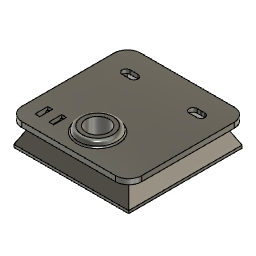
Lichtschranke Halterung (Autodesk Fusion 360 design; units mm, degrees)
Autodesk Fusion 360 part; units mm, degrees
sketch "Skizze1" plane through (0, 0, 0) normal (0, 0, 1) x (1, 0, 0)
  line L0 (0, 0) -> (43.5, 0)
  line L1 (43.5, 0) -> (43.5, 43)
  line L2 (43.5, 43) -> (0, 43)
  line L3 (0, 43) -> (0, 0)
  line L4 (-0.0245, 10) -> (43.5, 10) construction
  line L5 (21.75, 0) -> (21.75, 43) construction
  circle A0 centre (21.7377, 10) radius 4.35
  circle A1 centre (21.7377, 10) radius 7.35
  line L6 (-0.0245, 10) -> (43.5587, 10)
  line L7 (43.5587, 10) -> (43.5587, 8)
  line L8 (43.5587, 8) -> (-0.0245, 8)
  line L9 (-0.0245, 8) -> (-0.0245, 10)
  line L10 (43.5587, 12) -> (-0.0245, 12)
  line L11 (0, -23) -> (0, 20)
  line L12 (43.5, 20) -> (43.5, -23)
  line L13 (21.75, 0) -> (23.75, 0)
  line L14 (23.75, 0) -> (23.75, 43)
  line L15 (23.75, 43) -> (21.75, 43)
  line L16 (21.75, 43) -> (21.75, 0)
  line L17 (19.75, 0) -> (19.75, 43)
  line L18 (19.75, 43) -> (21.75, 43)
  line L19 (21.75, 0) -> (19.75, 0)
  dimension "d1" = 43.5
  dimension "d2" = 43
  dimension "d94" = 8.7
  dimension "d95" = 14.7
  dimension "d100" = 10
  dimension "d107" = 2
  dimension "d108" = 43.5833
  dimension "d109" = 2
  constraint horizontal L0
  constraint vertical L1
  constraint horizontal L2
  constraint vertical L3
  constraint coincident L0.start L3.end
  constraint midpoint L0 L5.start
  constraint midpoint L2 L5.end
  constraint concentric A0 A1
  constraint perpendicular L1 L4
  constraint horizontal L6
  constraint vertical L7
  constraint horizontal L8
  constraint vertical L9
  constraint symmetric L0.start L6 L11.end
  constraint symmetric L0.end L6 L12.start
  constraint symmetric L1.end L6 L12.end
  constraint symmetric L2.end L6 L11.start
  constraint symmetric L7.end L6 L10.start
  constraint symmetric L8.end L6 L10.end
  constraint horizontal L13
  constraint vertical L14
  constraint horizontal L15
  constraint vertical L16
  constraint symmetric L13.start L5 L16.end
  constraint symmetric L5 L13.end L17.start
  constraint symmetric L5 L14.end L17.end
  constraint symmetric L5 L15.end L16.start
  measures "d1" distance of L0.start L0.end
  measures "d2" distance of L0.start L2.end
  measures "d94" diameter of A0
  measures "d95" diameter of A1
  measures "d100" distance of L0.end L4.end
  measures "d107" distance of L4.start L8.end
  measures "d108" distance of L7.end L8.end
  measures "d109" distance of L5.start L13.end
extrude "Extrusion1" add sketch "Skizze1" along normal blind 1 contours L0 L3 A1 L8 L11 L17 | L0 A1 L16 L17 L19 | L3 A1 L6 L8 L11 | L0 A1 L13 L14 L16 | A0 A1 L16 L17 | A0 A1 L8 L17 | L3 A1 L6 L10 L11 | A0 A1 L6 L8 | L0 L1 A1 L8 L12 L14 | A0 A1 L14 L16 | A0 L8 L16 L17 | A0 L8 L17 | L2 L3 A1 L10 L11 L17 | A0 A1 L6 L10 | A0 L6 L8 L17 | A0 A1 L8 L14 | A0 L8 L14 L16 | L6 L8 L16 L17 | A0 A1 L10 L17 | A0 L6 L10 L17 | L1 A1 L6 L8 L12 | A0 A1 L6 L8 | A0 L8 L14 | L6 L8 L14 L16 | L6 L10 L16 L17 | L2 A1 L16 L17 L18 | A0 A1 L16 L17 | A0 L10 L17 | L1 A1 L6 L10 L12 | A0 A1 L6 L10 | A0 L6 L8 L14 | L6 L10 L14 L16 | A0 L10 L16 L17 | L2 A1 L14 L15 L16 | A0 A1 L14 L16 | L1 L2 A1 L10 L12 L14 | A0 A1 L10 L14 | A0 L6 L10 L14 | A0 L10 L14 L16 | A0 L10 L14
extrude "Extrusion2" add 1 faces at (29, 21, 1) along direction (0, 0, 1) blind 8
chamfer "Fase1" distance 4 distance2 8 4 edges at (21.75, 0, 9) (43.5, 21.5, 9) (21.75, 43, 9) (0, 21.5, 9) measured on face at (14.5, 28.6667, 9) measured on face at (14.5, 28.6667, 9) measured on face at (14.5, 28.6667, 9) measured on face at (14.5, 28.6667, 9)
sketch "Skizze2" plane through (0, 0, 9) normal (0, 0, 1) x (-1, 0, 0)
  line L0 (-39.5, -39) -> (-4, -39) construction
  line L1 (-4, -39) -> (-4, -4) construction
  line L2 (-4, -4) -> (-39.5, -4) construction
  line L3 (-39.5, -4) -> (-39.5, -39) construction
  line L4 (-39.5, -4) -> (-4, -39) construction
  line L5 (-4, -4) -> (-39.5, -39) construction
  line L6 (-44.5, -44) -> (1, -44)
  line L7 (1, -44) -> (1, 1)
  line L8 (1, 1) -> (-44.5, 1)
  line L9 (-44.5, 1) -> (-44.5, -44)
  dimension "d9" = 5
  constraint coincident L2.end L3.start
  constraint coincident L0.end L1.start
  constraint coincident L1.end L2.start
  constraint coincident L0.start L3.end
extrude "Extrusion3" add sketch "Skizze2" along normal blind 2
fillet "Abrundung1" radius 5 4 edges at (44.5, 44, 10) (-1, 44, 10) (-1, -1, 10) (44.5, -1, 10)
shell "Schale1" thickness 1.5 removed faces 1 at (29, 14.3333, 0)
sketch "Skizze7" plane through (0, 0, 11) normal (0, 0, 1) x (-1, 0, 0)
  arc A0 (-39.5, 1) -> (-44.5, -4) centre (-39.5, -4) ccw
  line L0 (-44.5, -4) -> (-44.5, -39)
  arc A1 (-44.5, -39) -> (-39.5, -44) centre (-39.5, -39) ccw
  line L1 (-39.5, -44) -> (-4, -44)
  arc A2 (-4, -44) -> (1, -39) centre (-4, -39) ccw
  line L2 (1, -39) -> (1, -4)
  arc A3 (1, -4) -> (-4, 1) centre (-4, -4) ccw
  line L3 (-4, 1) -> (-39.5, 1)
  line L4 (-6.25, -38) -> (-37.25, -38)
  line L5 (-37.25, -38) -> (-37.25, -18)
  line L6 (-37.25, -18) -> (-6.25, -18)
  line L7 (-6.25, -18) -> (-6.25, -38)
  line L8 (-21.75, -44) -> (-21.75, -32) construction
  circle A4 centre (-34.45, -35) radius 1.5
  circle A5 centre (-9.05, -35) radius 1.5
  line L9 (-4, -8.8) -> (-11.1, -8.8)
  line L10 (-11.1, -8.8) -> (-11.1, -4)
  line L11 (-11.1, -4) -> (-4, -4)
  line L12 (-4, -4) -> (-4, -8.8)
  line L13 (-5.8, -8.8) -> (-9.3, -8.8) construction
  line L14 (-9.3, -8.8) -> (-9.3, -4)
  line L15 (-9.3, -4) -> (-5.8, -4) construction
  line L16 (-5.8, -4) -> (-5.8, -8.8)
  arc A6 (-39.5, 1) -> (-44.5, -4) centre (-39.5, -4) ccw
  line L17 (-39.5, 1) -> (-4, 1)
  arc A7 (1, -4) -> (-4, 1) centre (-4, -4) ccw
  line L18 (1, -4) -> (1, -39)
  arc A8 (-4, -44) -> (1, -39) centre (-4, -39) ccw
  line L19 (-4, -44) -> (-39.5, -44)
  arc A9 (-44.5, -39) -> (-39.5, -44) centre (-39.5, -39) ccw
  line L20 (-44.5, -39) -> (-44.5, -4)
  line L21 (-39.5, -39) -> (-4, -39)
  line L22 (-4, -39) -> (-4, -4)
  line L23 (-4, -4) -> (-39.5, -4)
  line L24 (-39.5, -4) -> (-39.5, -39)
  circle A10 centre (-7.55, -35) radius 1.5
  circle A11 centre (-10.55, -35) radius 1.5
  circle A12 centre (-32.95, -35) radius 1.5
  circle A13 centre (-35.95, -35) radius 1.5
  line L25 (-32.9776, -36.4997) -> (-35.9499, -36.5)
  line L26 (-32.9776, -33.5003) -> (-35.9499, -33.5)
  line L27 (-7.5499, -36.5) -> (-10.55, -36.5)
  line L28 (-7.5501, -33.5) -> (-10.55, -33.5)
  dimension "d58" = 31
  dimension "d59" = 20
  dimension "d60" = 6
  dimension "d61" = 2.8
  dimension "d62" = 2.8
  dimension "d63" = 3
  dimension "d64" = 3
  dimension "d65" = 3
  dimension "d66" = 3
  dimension "d69" = 5
  dimension "d70" = 5
  dimension "d73" = 4.8
  dimension "d74" = 7.1
  dimension "d86" = 3.5
  dimension "d87" = 4.8
  dimension "d90" = 3
  dimension "d91" = 3
  dimension "d92" = 3
  dimension "d93" = 3
  constraint horizontal L4
  constraint vertical L5
  constraint horizontal L6
  constraint vertical L7
  constraint midpoint L1 L8.start
  constraint perpendicular L4 L8
  constraint midpoint L4 L8
  constraint horizontal L9
  constraint vertical L10
  constraint horizontal L11
  constraint vertical L12
  constraint horizontal L13
  constraint vertical L14
  constraint horizontal L15
  constraint vertical L16
  constraint coincident L9 L13.start
  constraint midpoint L9 L13
  constraint coincident A12 L25.start
  constraint coincident A13 L25.end
  constraint tangent A13 L25
  constraint coincident A12 L26.start
  constraint coincident A13 L26.end
  constraint tangent A13 L26
  constraint coincident A10 L27.start
  constraint coincident A11 L27.end
  constraint tangent A11 L27
  constraint coincident A10 L28.start
  constraint coincident A11 L28.end
  constraint tangent A11 L28
  measures "d58" distance of L4.start L4.end
  measures "d59" distance of L4.start L6.end
  measures "d60" distance of L1 L4
  measures "d61" distance of L5 A4.centre
  measures "d62" distance of L7 A5.centre
  measures "d63" distance of L4 A4.centre
  measures "d64" distance of L4 A5.centre
  measures "d65" diameter of A5
  measures "d66" diameter of A4
  measures "d69" distance of L3 L11
  measures "d70" distance of L2.end L12
  measures "d73" distance of L9.end L10.end
  measures "d74" distance of L9.start L9.end
  measures "d86" distance of L13.start L13.end
  measures "d87" distance of L13.end L14.end
  measures "d90" diameter of A10
  measures "d91" diameter of A11
  measures "d92" diameter of A12
  measures "d93" diameter of A13
extrude "Extrusion8" cut sketch "Skizze7" against normal blind 5 contours L7 A5 A10 | L7 A10 | L5 A13 | L5 A4 A13 | A5 A10 L27 | A4 A13 L25 | A5 A10 L28 | A5 A10 | A5 A10 A11 | A5 A11 L27 | A4 A13 L26 | A4 A12 A13 | A4 A13 | A4 A12 L25 | A5 A10 A11 | A5 A11 L28 | A5 A11 | A5 A11 | A4 A12 A13 | A4 A12 L26 | A4 A12 | A4 A12
extrude "Extrusion12" cut sketch "Skizze7" against normal blind 10 contours L9 L11 L12 L16 L22 L23 | L9 L10 L11 L14 L23
extrude "Extrusion13" cut sketch "Skizze1" along normal blind 13 contours A0 L8 L16 L17 | A0 L8 L17 | A0 L6 L8 L17 | A0 L8 L14 L16 | L6 L8 L16 L17 | A0 L6 L10 L17 | A0 L8 L14 | L6 L8 L14 L16 | L6 L10 L16 L17 | A0 L10 L17 | A0 L6 L8 L14 | L6 L10 L14 L16 | A0 L10 L16 L17 | A0 L6 L10 L14 | A0 L10 L14 L16 | A0 L10 L14
extrude "Extrusion14" add sketch "Skizze1" along normal blind 13 contours A0 A1 L16 L17 | A0 A1 L8 L17 | A0 A1 L6 L8 | A0 A1 L14 L16 | A0 A1 L6 L10 | A0 A1 L8 L14 | A0 A1 L10 L17 | A0 A1 L6 L8 | A0 A1 L16 L17 | A0 A1 L6 L10 | A0 A1 L14 L16 | A0 A1 L10 L14
sketch "Skizze11" plane through (43.5, 0, 0) normal (1, 0, 0) x (0, 1, 0)
  line L0 (43, 1) -> (0, 1)
  line L1 (0, 1) -> (0, 0)
  line L2 (0, 0) -> (43, 0)
  line L3 (43, 0) -> (43, 1)
  line L4 (4, 9) -> (-1, 9)
  line L5 (4, 9) -> (0, 1)
  line L6 (-1, 9) -> (0, 1)
  line L7 (39, 9) -> (43, 1)
  line L8 (44, 9) -> (39, 9)
  line L9 (44, 9) -> (43, 1)
  constraint coincident L4.end L6.start
  constraint coincident L0.end L1.start
  constraint coincident L8.start L9.start
  constraint coincident L0.start L3.end
extrude "Extrusion16" add sketch "Skizze1" along normal blind 10 contours L0 A1 L16 L17 L19 | L3 A1 L6 L8 L11 | L0 A1 L13 L14 L16 | L3 A1 L6 L10 L11 | L1 A1 L6 L8 L12 | L2 A1 L16 L17 L18 | L1 A1 L6 L10 L12 | L2 A1 L14 L15 L16
fillet "Abrundung5" radius 0.5 1 edges at (14.8851, 12.6579, 11)
fillet "Abrundung5" radius 1.5 1 edges at (14.8851, 7.3421, 13)
extrude "Extrusion15" cut sketch "Skizze11" against normal blind 32 contours L4 L5 L6 | L7 L8 L9
sketch "Skizze12" plane through (0, 44, 0) normal (0, 1, 0) x (-1, 0, 0)
  line L0 (-4, 9) -> (-4, 11)
  line L1 (-4, 11) -> (-39.5, 11)
  line L2 (-39.5, 11) -> (-39.5, 9)
  line L3 (-39.5, 9) -> (-4, 9)
  line L4 (-39.5, 9) -> (-44.5, 9)
  line L5 (-39.5, 9) -> (-43.5, 1)
  line L6 (-4, 9) -> (0, 1)
  line L7 (1, 9) -> (-4, 9)
  line L8 (1, 9) -> (0, 1)
  line L9 (-44.5, 9) -> (-43.5, 1)
  constraint coincident L7.start L8.start
  constraint coincident L6.end L8.end
  constraint coincident L4.end L9.start
  constraint coincident L5.end L9.end
extrude "Extrusion17" cut sketch "Skizze12" against normal blind 43 contours L4 L5 L9 | L6 L7 L8
chamfer "Fase2" distance 0.5 angle 45 2 edges at (10.2, 8, 10) (4.9, 8, 10)
equation "d74 = d86 + 1.8 mm + 1.8 mm"
equation "d87 = d73"
equation "d95 = d94 + ( 2 * 3 ) * 1 mm"
